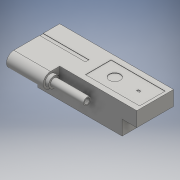
# Autodesk Inventor part: UCAM-DLI500TNBK
Saved by Autodesk Inventor 2016 (Build 200138000, 138)
## iProperties
Created: 2016-11-11
Part Number: UCAM-DLI500TNBK
Material: 一般
Document SubType Name: Modeling
Designer: Daisuke
Density: 1 g/cm^3
Appearance: 既定
Author: Daisuke
Autodesk Inventor part; units mm, degrees
ref_plane "YZ Plane" through (0, 0, 0) normal (1, 0, 0) x (0, 1, 0)
ref_plane "XZ Plane" through (0, 0, 0) normal (0, 1, 0) x (-1, 0, 0)
ref_plane "XY Plane" through (0, 0, 0) normal (0, 0, 1) x (1, 0, 0)
sketch "スケッチ1" plane through (0, 0, 0) normal (0, 0, 1) x (1, 0, 0)
  line L0 (0, 0) -> (62, 0)
  line L1 (62, 0) -> (62, 20)
  line L2 (62, 20) -> (0, 20)
  line L3 (0, 20) -> (0, 0)
  dimension "d0" = 62
  dimension "d1" = 20
  constraints: 8 end point, 2 parallel, 1 horizontal, 1 perpendicular
  measures "d0" distance of L2.end L1.end
  measures "d1" distance of L1.end L0.end
extrude "押し出し1" add sketch "スケッチ1" along normal blind 8
sketch "スケッチ2" plane through (0, 0, 0) normal (-1, 0, 0) x (0, 0, 1)
  line L0 (0, 0) -> (8, 0) projected
  line L1 (4, 0) -> (4, -1)
  line L2 (4, -1) -> (4, -5) construction
  circle A0 centre (4, -5) radius 4
  line L3 (8, 0) -> (8, -5)
  circle A1 centre (4, -5) radius 3
  dimension "d4" = 1
  dimension "d5" = 4
  dimension "d6" = 6
  constraints: 6 end point, 2 centre point, 2 coincident, 2 point on circle, 2 vertical, 1 midpoint, 1 tangent
  measures "d4" distance of L1.start L1.end
  measures "d5" distance of L1.end L2.end
  measures "d6" diameter of A1
extrude "押し出し2" add sketch "スケッチ2" against normal blind 20
sketch "スケッチ3" plane through (20, 0, 0) normal (1, 0, 0) x (0, 0, -1)
  arc A0 (-8, -5) -> (-4, -1) centre (-4, -5) ccw construction
  line L0 (0, 0) -> (-4, 0) construction
  line L1 (-4, 0) -> (-4, -5) construction
  line L2 (-4, -5) -> (0, -5) construction
  line L3 (0, -5) -> (0, 0) construction
  circle A1 centre (-4, -5) radius 3
  constraints: 8 end point, 2 parallel, 1 centre point, 1 coincident, 1 horizontal, 1 perpendicular
extrude "押し出し3" add sketch "スケッチ3" along normal blind 2 and the other way blind 10
sketch "スケッチ4" plane through (22, -5, 4) normal (1, 0, 0) x (0, 0, -1)
  circle A0 centre (0, 0) radius 2
  circle A1 centre (0, 0) radius 1.5
  point P0 (4, 5)
  dimension "d13" = 4
  dimension "d14" = 3
  constraints: 2 centre point, 1 coincident
  measures "d13" diameter of A0
  measures "d14" diameter of A1
extrude "押し出し4" add sketch "スケッチ4" along normal blind 18
sketch "スケッチ5" plane through (0, 0, 0) normal (0, 0, -1) x (-1, 0, 0)
  line L0 (0, 0) -> (-62, 0) construction
  line L1 (0, 0) -> (-8, 0) construction
  line L2 (-62, 0) -> (-54, 0) construction
  line L3 (-62, 20) -> (0, 20) projected
  line L4 (-8, 0) -> (-54, 0)
  line L5 (-54, 0) -> (-54, 20)
  line L6 (-54, 20) -> (-8, 20)
  line L7 (-8, 20) -> (-8, 0)
  dimension "d17" = 8
  dimension "d18" = 8
  constraints: 12 end point, 3 point on line, 2 parallel, 1 horizontal, 1 perpendicular
  measures "d17" distance of L0.start L1.end
  measures "d18" distance of L0.end L2.end
extrude "押し出し5" add sketch "スケッチ5" along normal blind 8
chamfer "面取り1" distance 3 distance2 8 1 edges at (31, 20, -8) measured on face at (23.3333, 6.6667, -8)
sketch "スケッチ6" plane through (0, 0, -8) normal (0, 0, -1) x (-1, 0, 0)
  line L0 (-54, 17) -> (-8, 17) construction
  line L1 (-8, 17) -> (-9.5, 17) construction
  line L2 (-9.5, 17) -> (-9.5, 16) construction
  line L3 (-9.5, 16) -> (-8, 16) construction
  line L4 (-8, 16) -> (-8, 17) construction
  line L5 (-9.5, 16) -> (-19, 16)
  line L6 (-19, 16) -> (-19, 10)
  line L7 (-19, 10) -> (-9.5, 10)
  line L8 (-9.5, 10) -> (-9.5, 16)
  point P0 (0, 0)
  dimension "d26" = 9.5
  dimension "d27" = 6
  dimension "d28" = 1.5
  dimension "d29" = 1
  constraints: 16 end point, 4 parallel, 2 horizontal, 2 perpendicular
  measures "d26" distance of L7.end L6.end
  measures "d27" distance of L6.end L5.end
  measures "d28" distance of L0.end L1.end
  measures "d29" distance of L3.end L0.end
extrude "押し出し6" add sketch "スケッチ6" along normal blind 1
sketch "スケッチ7" plane through (0, 0, 8) normal (0, 0, 1) x (1, 0, 0)
  line L0 (0, 0) -> (0, 9) construction
  line L1 (0, 20) -> (0, 0) construction
  line L2 (0, 9) -> (25, 9)
  line L3 (25, 9) -> (25, 11)
  line L4 (25, 11) -> (0, 11)
  line L5 (0, 11) -> (0, 9)
  line L6 (20, 0) -> (62, 0) construction
  line L7 (62, 0) -> (60.5, 0) construction
  line L8 (60.5, 0) -> (60.5, 3) construction
  line L9 (60.5, 3) -> (62, 3) construction
  line L10 (62, 3) -> (62, 0) construction
  line L11 (60.5, 3) -> (31, 3)
  line L12 (31, 3) -> (31, 17)
  line L13 (31, 17) -> (60.5, 17)
  line L14 (60.5, 17) -> (60.5, 3)
  dimension "d32" = 9
  dimension "d33" = 25
  dimension "d34" = 2
  dimension "d37" = 1.5
  dimension "d38" = 3
  dimension "d39" = 29.5
  dimension "d40" = 14
  constraints: 26 end point, 6 parallel, 3 horizontal, 3 perpendicular, 1 point on line
  measures "d32" distance of L0.start L0.end
  measures "d33" distance of L4.end L3.end
  measures "d34" distance of L3.end L2.end
  measures "d37" distance of L8.end L9.end
  measures "d38" distance of L7.end L8.end
  measures "d39" distance of L12.end L13.end
  measures "d40" distance of L11.end L12.end
extrude "押し出し8" cut sketch "スケッチ7" against normal blind 0.2
sketch "スケッチ9" plane through (0, 0, 7.8) normal (0, 0, 1) x (1, 0, 0)
  line L0 (31, 3) -> (31, 17) construction
  line L1 (31, 10) -> (40, 10) construction
  circle A0 centre (40, 10) radius 3
  line L2 (60.5, 17) -> (60.5, 3) construction
  line L3 (60.5, 10) -> (53, 10) construction
  line L4 (52.25, 9.5) -> (53.75, 9.5)
  line L5 (53.75, 9.5) -> (53.75, 10.5)
  line L6 (53.75, 10.5) -> (52.25, 10.5)
  line L7 (52.25, 10.5) -> (52.25, 9.5)
  line L8 (52.25, 9.5) -> (53.75, 10.5) construction
  line L9 (53.75, 9.5) -> (52.25, 10.5) construction
  point P0 (0, 0)
  dimension "d43" = 9
  dimension "d44" = 6
  dimension "d45" = 7.5
  dimension "d46" = 1.5
  dimension "d47" = 1
  constraints: 16 end point, 4 midpoint, 3 horizontal, 2 parallel, 1 centre point, 1 coincident, 1 perpendicular
  measures "d43" distance of L1.start L1.end
  measures "d44" diameter of A0
  measures "d45" distance of L3.start L3.end
  measures "d46" distance of L6.end L5.end
  measures "d47" distance of L5.end L4.end
extrude "押し出し9" cut sketch "スケッチ9" against normal blind 0.3
thread "ねじ1" size "M3x0.5" class "6H" standard "ANSI Metric M Profile" full length
